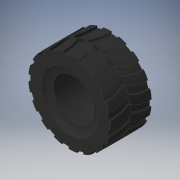
# Autodesk Inventor part: llanta2
Saved by Autodesk Inventor 2017 (Build 210142000, 142)
## iProperties
Created: 2016-09-09
Part Number: llanta2
Material: Generic
Document SubType Name: Modeling
Designer: santiago.solorzano
Density: 1 g/cm^3
Appearance: Goma - Negro
Author: santiago.solorzano
Autodesk Inventor part; units mm, degrees
note: some values were not read from the file. Chosen so that the rebuilt part matches the saved one: direction of "Emboss2".
ref_plane "YZ Plane" through (0, 0, 0) normal (1, 0, 0) x (0, 1, 0)
ref_plane "XY Plane" through (0, 0, 0) normal (0, 0, 1) x (1, 0, 0)
sketch "Sketch1" plane through (0, 0, 0) normal (0, 0, 1) x (1, 0, 0)
  circle A0 centre (0, 0) radius 61
  dimension "d0" = 122
  constraints: 1 centre point, 1 coincident
  measures "d0" diameter of A0
extrude "Extrusion1" add sketch "Sketch1" along normal blind 61
sketch "Sketch3" plane through (0, 0, 0) normal (0, 0, -1) x (-1, 0, 0)
  circle A0 centre (0, 0) radius 42
  dimension "d3" = 84
  constraints: 1 centre point, 1 coincident
  measures "d3" diameter of A0
extrude "Extrusion2" cut sketch "Sketch3" against normal blind 6
sketch "Sketch4" plane through (0, 0, 6) normal (0, 0, -1) x (-1, 0, 0)
  circle A0 centre (0, 0) radius 30.5
  dimension "d6" = 61
  constraints: 1 centre point, 1 coincident
  measures "d6" diameter of A0
extrude "Extrusion3" cut sketch "Sketch4" against normal blind 49
sketch "Sketch5" plane through (0, 0, 61) normal (0, 0, 1) x (1, 0, 0)
  circle A0 centre (0, 0) radius 42
  dimension "d9" = 84
  constraints: 1 centre point, 1 coincident
  measures "d9" diameter of A0
extrude "Extrusion4" cut sketch "Sketch5" against normal blind 6
fillet "Fillet1" radius 14 1 edges at (42, 0, 6)
fillet "Fillet2" radius 14 1 edges at (-42, 0, 55)
ref_plane "Work Plane3" through (0, 61, 0) normal (0, 1, 0) x (-1, 0, 0)
sketch "Sketch8" plane through (0, 61, 0) normal (0, 1, 0) x (-1, 0, 0)
  arc A0 (0, 61) -> (7, 30.5) centre (56.9216, 58.0107) ccw
  arc A1 (10, 61) -> (17, 30.5) centre (66.9216, 58.0107) ccw
  line L0 (17, 30.5) -> (27, 30.5)
  arc A2 (17, 30.5) -> (10, 0) centre (66.9216, 2.9893) ccw
  arc A3 (27, 30.5) -> (20, 0) centre (76.9216, 2.9893) ccw
  line L1 (7, 30.5) -> (17, 30.5)
  line L2 (10, 0) -> (20, 0)
  line L3 (10, 61) -> (0, 61)
  line L4 (61, 61) -> (-61, 61) projected
  circle A4 centre (5, 5.7152) radius 2
  circle A5 centre (7.794, 21.0592) radius 2
  circle A6 centre (21.366, 37.2484) radius 2
  circle A7 centre (17, 51.8584) radius 2
  point P0 (0, 0)
  dimension "d36" = 10
  dimension "d37" = 10
  dimension "d38" = 10
  dimension "d39" = 10
  dimension "d63" = 4
  dimension "d64" = 4
  dimension "d65" = 4
  dimension "d66" = 4
  constraints: 8 centre point, 8 end point, 8 point on circle, 2 horizontal, 1 collinear
  measures "d36" distance of L1.start L0.start
  measures "d37" distance of L3.start L3.end
  measures "d38" distance of L0.start L0.end
  measures "d39" distance of L2.start L2.end
  measures "d63" diameter of A4
  measures "d64" diameter of A5
  measures "d65" diameter of A6
  measures "d66" diameter of A7
emboss "Emboss2" sketch "Sketch8" operation cut depth 3 direction (0, -1, 0) contours L3 A1 L1 A0 | L0 A3 L2 A2
pattern_circular "Circular Pattern1" count 17 over 360 about axis through (0, 0, 0) along (0, 0, 1) of "Emboss2"
body "Solid1"
